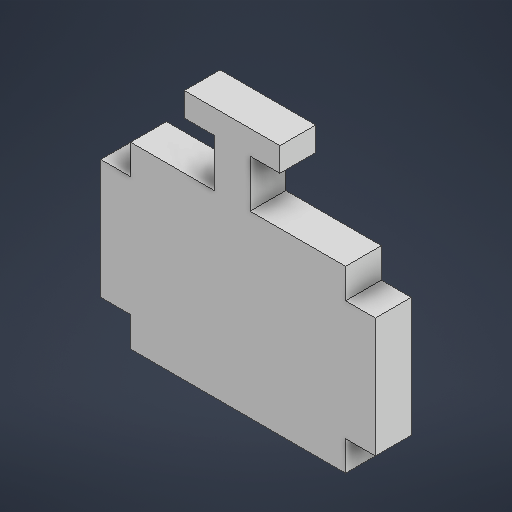
# Autodesk Inventor part: Spring_holder
Saved by Autodesk Inventor 2027 (Build 310192000, 192)
## iProperties
Created: 2026-05-09
Part Number: Spring_holder
Material: Generic
Document SubType Name: Modeling
Designer: alexy
Density: 1 g/cm^3
Appearance: Default
Author: alexy
Autodesk Inventor part; units mm, degrees
ref_plane "YZ Plane" through (0, 0, 0) normal (1, 0, 0) x (0, 1, 0)
ref_plane "XZ Plane" through (0, 0, 0) normal (0, 1, 0) x (-1, 0, 0)
ref_plane "XY Plane" through (0, 0, 0) normal (0, 0, 1) x (1, 0, 0)
sketch "Sketch1" plane through (0, 0, 0) normal (0, 0, 1) x (1, 0, 0)
  line L0 (0, 0) -> (18, 0)
  line L1 (18, 0) -> (18, 15)
  line L2 (18, 15) -> (0, 15)
  line L3 (0, 15) -> (0, 0)
  line L4 (20.5, 12.5) -> (18, 12.5)
  line L5 (18, 12.5) -> (18, 2.5)
  line L6 (18, 2.5) -> (20.5, 2.5)
  line L7 (20.5, 2.5) -> (20.5, 12.5)
  line L8 (20.5, 12.5) -> (18, 2.5) construction
  line L9 (18, 12.5) -> (20.5, 2.5) construction
  line L10 (-2.5, 12.5) -> (0, 12.5)
  line L11 (0, 12.5) -> (0, 2.5)
  line L12 (0, 2.5) -> (-2.5, 2.5)
  line L13 (-2.5, 2.5) -> (-2.5, 12.5)
  line L14 (-2.5, 12.5) -> (0, 2.5) construction
  line L15 (0, 12.5) -> (-2.5, 2.5) construction
  line L16 (7, 15) -> (7, 19)
  line L17 (7, 19) -> (4.5, 19)
  line L18 (4.5, 19) -> (4.5, 21)
  line L19 (4.5, 21) -> (12.5, 21)
  line L20 (12.5, 21) -> (12.5, 19)
  line L21 (12.5, 19) -> (10, 19)
  line L22 (10, 19) -> (10, 15)
  point P0 (19.25, 7.5)
  point P1 (-1.25, 7.5)
  point P2 (18, 7.5)
  point P3 (0, 7.5)
  point P4 (0, 12.5)
  dimension "d0" = 18
  dimension "d1" = 15
  dimension "d2" = 2.5
  dimension "d3" = 2.5
  dimension "d4" = 10
  dimension "d5" = 4
  dimension "d6" = 2.5
  dimension "d7" = 2
  dimension "d8" = 8
  dimension "d9" = 2
  dimension "d10" = 2.5
  dimension "d11" = 7
  constraints: 46 end point, 7 perpendicular, 7 point on line, 6 midpoint, 6 parallel, 3 horizontal, 2 horizontal alignment, 1 vertical
  measures "d0" distance of L2.end L1.end
  measures "d1" distance of L0.end L1.end
  measures "d2" distance of L5.end L6.end
  measures "d3" distance of L11.end L12.end
  measures "d4" distance of L12.end L10.start
  measures "d5" distance of L16.start L16.end
  measures "d6" distance of L16.end L17.end
  measures "d7" distance of L17.end L18.end
  measures "d8" distance of L18.end L19.end
  measures "d9" distance of L19.end L20.end
  measures "d10" distance of L20.end L21.end
  measures "d11" distance from line of L2.end L16
extrude "Extrusion1" add sketch "Sketch1" along normal blind 3
body "Solid1"
